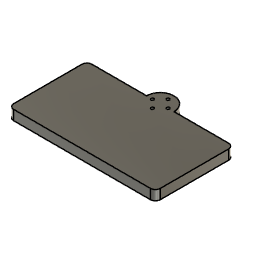
_Arm base.2ffd8a9a-10d5-4f2f-9273-e72e92dafab5 (Autodesk Fusion 360 design; units mm, degrees)
Autodesk Fusion 360 part; units mm, degrees
sketch "Sketch1" plane through (0, 0, 0) normal (0, 0, 1) x (1, 0, 0)
  line L0 (75, 40) -> (-75, 40)
  line L1 (-75, 40) -> (-75, -40)
  line L2 (-75, -40) -> (75, -40)
  line L3 (75, -40) -> (75, 40)
  line L4 (75, 40) -> (-75, -40) construction
  line L5 (-75, 40) -> (75, -40) construction
  dimension "d1" = 150
  dimension "d2" = 80
  constraint horizontal L0
  constraint perpendicular L0 L1
  constraint parallel L0 L2
  constraint parallel L1 L3
  constraint coincident L4 origin
  constraint coincident L5 origin
  measures "d1" distance of L1.end L2.end
  measures "d2" distance of L0.end L1.end
extrude "Extrude1" add sketch "Sketch1" along normal blind 10
sketch "Sketch2" plane through (0, 0, 0) normal (0, 0, 1) x (1, 0, 0)
  circle A0 centre (0, 40) radius 14
  dimension "d10" = 28
  measures "d10" diameter of A0
extrude "Extrude2" add sketch "Sketch2" along normal blind 10
sketch "Sketch3" plane through (0, 0, 0) normal (0, 0, 1) x (1, 0, 0)
  circle A0 centre (0, 40) radius 11
  dimension "d7" = 22
  measures "d7" diameter of A0
extrude "Extrude3" cut sketch "Sketch3" along normal blind 8
fillet "Fillet1" radius 5 4 edges at (75, -40, 5) (75, 40, 5) (-75, -40, 5) (-75, 40, 5)
sketch "Sketch4" plane through (0, 0, 8) normal (0, 0, -1) x (1, 0, 0)
  circle A0 centre (0, -32) radius 1.5
  circle A1 centre (0, -48) radius 1.5
  circle A2 centre (-8, -40) radius 1.5
  circle A3 centre (8, -40) radius 1.5
  circle A4 centre (0, -40) radius 11
  dimension "d13" = 3
  dimension "d14" = 3
  dimension "d15" = 3
  dimension "d16" = 3
  measures "d13" diameter of A0
  measures "d14" diameter of A1
  measures "d15" diameter of A2
  measures "d16" diameter of A3
extrude "Extrude4" cut sketch "Sketch4" against normal blind 2 contours A0 | A1 | A2 | A3
